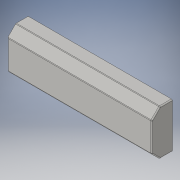
# Autodesk Inventor part: batt_cap
Saved by Autodesk Inventor 2016 (Build 200138000, 138)
## iProperties
Created: 2016-02-15
Part Number: batt_cap
Material: Glass
Document SubType Name: Modeling
Designer: jforce
Density: 2.18 g/cm^3
Appearance: Clear
Author: jforce
Autodesk Inventor part; units mm, degrees
ref_plane "YZ Plane" through (0, 0, 0) normal (1, 0, 0) x (0, 1, 0)
ref_plane "XZ Plane" through (0, 0, 0) normal (0, 1, 0) x (-1, 0, 0)
ref_plane "XY Plane" through (0, 0, 0) normal (0, 0, 1) x (1, 0, 0)
sketch "Sketch1" plane through (0, 0, 0) normal (0, 0, 1) x (1, 0, 0)
  line L0 (0, 0) -> (70, 0)
  line L1 (70, 0) -> (70, 22)
  line L2 (70, 22) -> (0, 22)
  line L3 (0, 22) -> (0, 0)
  dimension "d0" = 70
  dimension "d1" = 22
  constraints: 8 end point, 2 parallel, 1 horizontal, 1 perpendicular
  measures "d0" distance of L2.end L1.end
  measures "d1" distance of L1.end L0.end
extrude "Extrusion1" add sketch "Sketch1" along normal blind 10
chamfer "Chamfer1" distance 4 angle 45 2 edges at (35, 22, 10) (35, 0, 10)
fillet "Fillet1" radius 0.5 12 edges at (35, 22, 6) (35, 18, 10) (70, 20, 8) (70, 22, 3) (70, 11, 10) (70, 2, 8) (70, 0, 3) (35, 4, 10) (0, 11, 10) (0, 2, 8) (0, 0, 3) (35, 0, 6)
body "Solid1"
